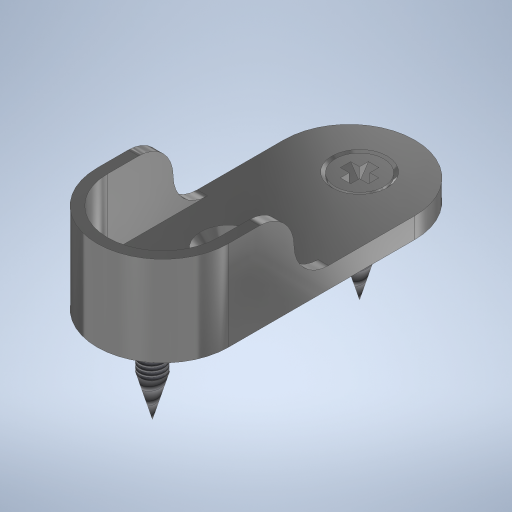
# Autodesk Inventor part: Fixture for the Oval Bar
Saved by Autodesk Inventor 2024 (Build 280153000, 153)
## iProperties
Created: 2015-03-09
Part Number: Fixture for the Oval Bar
Material: Steel
Document SubType Name: Modeling
Designer: SauliusD
Mass: 22.3457 g
Surface Area: 28.7197 cm^2
Volume: 2.84659 cm^3
Density: 7.85 g/cm^3
Appearance: Plate
Author: SauliusD
Autodesk Inventor part; units mm, degrees
ref_plane "YZ Plane" through (0, 0, 0) normal (1, 0, 0) x (0, 1, 0)
ref_plane "XZ Plane" through (0, 0, 0) normal (0, 1, 0) x (-1, 0, 0)
ref_plane "XY Plane" through (0, 0, 0) normal (0, 0, 1) x (1, 0, 0)
sketch "Sketch1" plane through (0, 0, 0) normal (0, 0, 1) x (1, 0, 0)
  line L0 (0, -13.5) -> (0, 13.5) construction
  line L1 (8, -13.5) -> (8, 13.5)
  line L2 (-8, 13.5) -> (-8, -13.5)
  arc A0 (-8, -13.5) -> (8, -13.5) centre (0, -13.5) ccw
  arc A1 (8, 13.5) -> (-8, 13.5) centre (0, 13.5) ccw
  line L3 (-9.5, 13.5) -> (-9.5, -13.5)
  arc A2 (-9.5, -13.5) -> (9.5, -13.5) centre (0, -13.5) ccw
  line L4 (9.5, -13.5) -> (9.5, 13.5)
  arc A3 (9.5, 13.5) -> (-9.5, 13.5) centre (0, 13.5) ccw
  line L5 (0, 23) -> (-20.3144, 23) construction
  line L6 (0, -23) -> (-17.7567, -23) construction
  point P0 (0, 0)
  point P1 (0, 15)
  point P2 (0, -4)
  point P3 (0, -15)
  dimension "d2" = 1.5
  dimension "d3" = 19
  dimension "d6" = 46
  dimension "d7" = 8
  dimension "d8" = 8
  dimension "d13" = 11
  constraints: 16 end point, 10 point on circle, 6 tangent, 4 centre point, 3 point on line, 2 horizontal, 2 parallel, 1 midpoint, 1 vertical, 3 other
  measures "d2" radial gap between concentric circles of A1 A3
  measures "d3" distance between parallel lines of L4 L3
  measures "d6" distance between parallel lines of L6 L5
  measures "d7" distance from line of L6 point (0, -15)
  measures "d8" distance from line of L5 point (0, 15)
  measures "d13" distance of point (0, -15) point (0, -4)
extrude "Extrusion1" add sketch "Sketch1" along normal blind 3 contours A0 L2 A1 L1 | A3 L4 A2 L3
extrude "Extrusion2" add sketch "Sketch1" along normal blind 13
sketch "Sketch2" plane through (8, -13.5, 3) normal (-1, 0, 0) x (0, 0, 1)
  line L0 (-3, 36.5) -> (10, 36.5) projected
  line L1 (10, 0) -> (10, 0) projected
  line L2 (10, 0) -> (10, 27) projected
  line L3 (10, 27) -> (10, 27) projected
  line L4 (10, 27) -> (10, 0) projected
  line L5 (10, 27) -> (10, 0) projected
  line L6 (10, 0) -> (10, 0) projected
  line L7 (10, 0) -> (10, 27) projected
  line L8 (10, 27) -> (10, 27) projected
  line L9 (0, 0) -> (0, 0) projected
  line L10 (0, 0) -> (0, 27) projected
  line L11 (0, 27) -> (0, 27) projected
  line L12 (0, 27) -> (0, 0) projected
  line L13 (0, 9.5) -> (10, 9.5)
  line L14 (10, 9.5) -> (10, 36.5)
  line L15 (10, 36.5) -> (0, 36.5)
  line L16 (0, 36.5) -> (0, 9.5)
  point P0 (-3, 13.5)
  point P1 (-3, 9.5)
  constraints: 8 end point, 2 parallel, 2 point on line, 1 horizontal, 1 perpendicular
extrude "Extrusion3" cut sketch "Sketch2" along normal through all both and the other way through all
fillet "Fillet1" radius 5 4 edges at (8.75, -4, 13) (8.75, -4, 3) (-8.75, -4, 13) (-8.75, -4, 3)
sketch "Sketch3" plane through (0, 0, 3) normal (0, 0, 1) x (1, 0, 0)
  point P0 (0, 0)
  point P1 (0, 15)
  point P2 (0, -4)
  point P3 (0, -15)
hole "Hole1" at (0, 15, 3) at (0, -4, 3) at (0, -15, 3) direction (0, 0, -1) diameter 5 depth 8 tip angle 118 countersink diameter 8 countersink angle 90
sketch "Sketch4" plane through (0, 0, 0) normal (1, 0, 0) x (0, 1, 0)
  line L0 (15, 2.895) -> (18.5, 2.895)
  line L1 (18.5, 2.895) -> (18.5, 2.495)
  line L2 (18.5, 2.495) -> (16.075, 0.07)
  line L3 (16.075, 0.07) -> (16.075, -2.53)
  line L4 (16.075, -2.53) -> (16.75, -2.7757)
  line L5 (16.75, -2.7757) -> (16.75, -7.002)
  line L6 (16.75, -7.002) -> (15, -13.105)
  line L7 (15, -13.105) -> (15, 2.895)
  line L8 (15, -18.326) -> (15, 18.221) projected
  line L9 (17.5, 1.5) -> (19, 3) projected
  point P0 (0, 0)
  dimension "d24" = 7
  dimension "d25" = 45
  dimension "d26" = 16
  dimension "d27" = 2.6
  dimension "d28" = 110
  dimension "d29" = 2.15
  dimension "d30" = 3.5
  dimension "d31" = 0.4
  dimension "d32" = 16
  constraints: 16 end point, 3 parallel, 1 collinear, 1 perpendicular
  measures "d24" diameter of L1 L7
  measures "d25" angle of L0 L2
  measures "d26" angle of L7 L6
  measures "d27" distance of L2.end L3.end
  measures "d28" angle of L4 L3
  measures "d29" diameter of L3 L7
  measures "d30" diameter of L5 L7
  measures "d31" distance of L0.end L1.end
  measures "d32" distance of L6.end L0.start
revolve "Revolution1" add sketch "Sketch4" angle 360 about axis through (0, 15, -13.105) along (0, 0, 1) separate body
thread "Thread1" size "M3.5x0.6" class "6g" standard "ANSI Metric M Profile" full length
thread "Thread2" size "R 4" standard "ISO Taper" full length
sketch "Sketch6" plane through (0, 0, 0) normal (1, 0, 0) x (0, 1, 0)
  line L0 (11.5, 2.895) -> (18.5, 2.895) projected
  line L1 (17.0355, 2.895) -> (15.75, 0.9703)
  line L2 (15.75, 0.9703) -> (14.25, 0.9703)
  line L3 (14.25, 0.9703) -> (12.9645, 2.895)
  line L4 (17.0355, 2.895) -> (12.9645, 2.895)
  line L5 (15, -2.6) -> (15, 15.6) projected
  point P0 (0, 0)
  dimension "d48" = 1.5
  constraints: 8 end point, 2 point on line, 1 collinear, 1 parallel, 1 other
  measures "d48" distance of L1.end L2.end
extrude "Extrusion4" cut sketch "Sketch6" along normal mid plane 1.5 bodies 2
pattern_circular "Circular Pattern1" count 2 over 90 about axis through (0, 15, -1) along (0, 0, 1) of "Extrusion4" bodies 2
sketch "Sketch7" plane through (-0.75, 15.75, 0.9703) normal (0, 0, 1) x (1, 0, 0)
  circle A0 centre (0.75, -0.75) radius 1.075 projected
  circle A1 centre (0.75, -0.75) radius 0.5
  point P0 (0.75, -15.75)
  dimension "d52" = 1
  constraints: 1 centre point, 1 coincident
  measures "d52" diameter of A1
extrude "Extrusion5" add sketch "Sketch7" against normal blind 10 separate body contours A1
pattern_linear "Rectangular Pattern1" count 2 spacing 30 along (0, -1, 0) bodies 2
pattern_linear "Rectangular Pattern2" count 2 spacing 30 along (0, -1, 0) bodies 3
equation "\"d16\" = -0.5 * d9 + 0.5 * d11"
equation "\"d24\" = d33"
equation "\"d27\" = d34"
equation "\"d29\" = d35"
equation "\"d30\" = d36"
equation "\"d32\" = d37"
equation "\"d33\" = 7"
equation "\"d34\" = 2.6"
equation "\"d35\" = 2.15"
equation "\"d36\" = 3.5"
equation "\"d37\" = 16"
equation "\"d9\" = 3"
equation "\"d11\" = 13"
